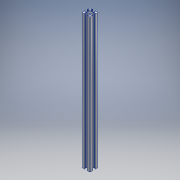
# Autodesk Inventor part: 2020 Extrusion - Double Z motor - Bed X
Saved by Autodesk Inventor 2016 (Build 200138000, 138)
## iProperties
Created: 2017-02-04
Part Number: 2020 Extrusion - Double Z motor - Bed X
Material: Aluminum 6061
Document SubType Name: Modeling
Designer: Scott
Mass: 170.679 g
Surface Area: 599.363 cm^2
Volume: 63.2146 cm^3
Density: 2.7 g/cm^3
Appearance: Aluminum - Flat
Author: Scott
Autodesk Inventor part; units mm, degrees
ref_plane "YZ Plane" through (0, 0, 0) normal (1, 0, 0) x (0, 1, 0)
ref_plane "XZ Plane" through (0, 0, 0) normal (0, 1, 0) x (-1, 0, 0)
ref_plane "XY Plane" through (0, 0, 0) normal (0, 0, 1) x (1, 0, 0)
sketch "Sketch1" plane through (0, 0, 0) normal (0, 0, 1) x (1, 0, 0)
  line L0 (-8, -10) -> (-3.2, -10)
  arc A0 (-10, -8) -> (-8, -10) centre (-8, -8) ccw
  line L1 (3.2, -10) -> (8, -10)
  line L2 (-8, 10) -> (-3.2, 10)
  line L3 (3.2, 10) -> (8, 10)
  line L4 (-10, 8) -> (-10, 3.2)
  arc A1 (-8, 10) -> (-10, 8) centre (-8, 8) ccw
  line L5 (-10, -3.2) -> (-10, -8)
  line L6 (10, 8) -> (10, 3.2)
  arc A2 (10, 8) -> (8, 10) centre (8, 8) ccw
  line L7 (10, -3.2) -> (10, -8)
  arc A3 (8, -10) -> (10, -8) centre (8, -8) ccw
  circle A4 centre (0, 0) radius 2.6
  line L8 (8.65, 4.6) -> (8.65, 3.2)
  line L9 (8.65, -3.2) -> (8.65, -4.6)
  arc A5 (8.15, -5.1) -> (8.65, -4.6) centre (8.15, -4.6) ccw
  arc A6 (8.65, 4.6) -> (8.15, 5.1) centre (8.15, 4.6) ccw
  line L10 (3.9, 2.0109) -> (3.9, -2.0109)
  arc A7 (4.4858, 3.4251) -> (3.9, 2.0109) centre (5.9, 2.0109) ccw
  line L11 (8.65, 3.2) -> (10, 3.2)
  line L12 (8.65, -3.2) -> (10, -3.2)
  line L13 (6.3678, -5.1) -> (8.15, -5.1)
  arc A8 (6.0142, -4.9536) -> (6.3678, -5.1) centre (6.3678, -4.6) ccw
  line L14 (6.3678, 5.1) -> (8.15, 5.1)
  arc A9 (6.3678, 5.1) -> (6.0142, 4.9536) centre (6.3678, 4.6) ccw
  line L15 (4.4858, 3.4251) -> (6.0142, 4.9536)
  line L16 (4.4858, -3.4251) -> (6.0142, -4.9536)
  arc A10 (3.9, -2.0109) -> (4.4858, -3.4251) centre (5.9, -2.0109) ccw
  line L17 (-4.6, 8.65) -> (-3.2, 8.65)
  line L18 (3.2, 8.65) -> (4.6, 8.65)
  arc A11 (5.1, 8.15) -> (4.6, 8.65) centre (4.6, 8.15) ccw
  arc A12 (-4.6, 8.65) -> (-5.1, 8.15) centre (-4.6, 8.15) ccw
  line L19 (-2.0109, 3.9) -> (2.0109, 3.9)
  arc A13 (-3.4251, 4.4858) -> (-2.0109, 3.9) centre (-2.0109, 5.9) ccw
  line L20 (-3.2, 8.65) -> (-3.2, 10)
  line L21 (3.2, 8.65) -> (3.2, 10)
  line L22 (5.1, 6.3678) -> (5.1, 8.15)
  arc A14 (4.9536, 6.0142) -> (5.1, 6.3678) centre (4.6, 6.3678) ccw
  line L23 (-5.1, 6.3678) -> (-5.1, 8.15)
  arc A15 (-5.1, 6.3678) -> (-4.9536, 6.0142) centre (-4.6, 6.3678) ccw
  line L24 (-3.4251, 4.4858) -> (-4.9536, 6.0142)
  line L25 (3.4251, 4.4858) -> (4.9536, 6.0142)
  arc A16 (2.0109, 3.9) -> (3.4251, 4.4858) centre (2.0109, 5.9) ccw
  line L26 (-8.65, -4.6) -> (-8.65, -3.2)
  line L27 (-8.65, 3.2) -> (-8.65, 4.6)
  arc A17 (-8.15, 5.1) -> (-8.65, 4.6) centre (-8.15, 4.6) ccw
  arc A18 (-8.65, -4.6) -> (-8.15, -5.1) centre (-8.15, -4.6) ccw
  line L28 (-3.9, -2.0109) -> (-3.9, 2.0109)
  arc A19 (-4.4858, -3.4251) -> (-3.9, -2.0109) centre (-5.9, -2.0109) ccw
  line L29 (-8.65, -3.2) -> (-10, -3.2)
  line L30 (-8.65, 3.2) -> (-10, 3.2)
  line L31 (-6.3678, 5.1) -> (-8.15, 5.1)
  arc A20 (-6.0142, 4.9536) -> (-6.3678, 5.1) centre (-6.3678, 4.6) ccw
  line L32 (-6.3678, -5.1) -> (-8.15, -5.1)
  arc A21 (-6.3678, -5.1) -> (-6.0142, -4.9536) centre (-6.3678, -4.6) ccw
  line L33 (-4.4858, -3.4251) -> (-6.0142, -4.9536)
  line L34 (-4.4858, 3.4251) -> (-6.0142, 4.9536)
  arc A22 (-3.9, 2.0109) -> (-4.4858, 3.4251) centre (-5.9, 2.0109) ccw
  line L35 (4.6, -8.65) -> (3.2, -8.65)
  line L36 (-3.2, -8.65) -> (-4.6, -8.65)
  arc A23 (-5.1, -8.15) -> (-4.6, -8.65) centre (-4.6, -8.15) ccw
  arc A24 (4.6, -8.65) -> (5.1, -8.15) centre (4.6, -8.15) ccw
  line L37 (2.0109, -3.9) -> (-2.0109, -3.9)
  arc A25 (3.4251, -4.4858) -> (2.0109, -3.9) centre (2.0109, -5.9) ccw
  line L38 (3.2, -8.65) -> (3.2, -10)
  line L39 (-3.2, -8.65) -> (-3.2, -10)
  line L40 (-5.1, -6.3678) -> (-5.1, -8.15)
  arc A26 (-4.9536, -6.0142) -> (-5.1, -6.3678) centre (-4.6, -6.3678) ccw
  line L41 (5.1, -6.3678) -> (5.1, -8.15)
  arc A27 (5.1, -6.3678) -> (4.9536, -6.0142) centre (4.6, -6.3678) ccw
  line L42 (3.4251, -4.4858) -> (4.9536, -6.0142)
  line L43 (-3.4251, -4.4858) -> (-4.9536, -6.0142)
  arc A28 (-2.0109, -3.9) -> (-3.4251, -4.4858) centre (-2.0109, -5.9) ccw
  dimension "d0" = 0.5
  dimension "d1" = 2
  dimension "d2" = 5.2
  dimension "d3" = 45
  dimension "d4" = 45
  dimension "d5" = 45
  dimension "d6" = 90
  dimension "d7" = 90
  dimension "d8" = 45
  dimension "d9" = 45
  dimension "d10" = 90
  dimension "d11" = 90
  dimension "d12" = 90
  dimension "d13" = 90
  dimension "d14" = 90
  dimension "d15" = 90
  dimension "d16" = 90
  dimension "d17" = 90
  dimension "d18" = 90
  dimension "d19" = 90
  dimension "d20" = 90
  dimension "d21" = 90
  dimension "d22" = 90
  dimension "d23" = 90
  dimension "d24" = 1.35
  dimension "d25" = 4.9
  dimension "d26" = 6.1
  dimension "d27" = 6.8
  dimension "d28" = 13.2
  dimension "d29" = 13.9
  dimension "d30" = 15.1
  dimension "d31" = 18.65
  dimension "d32" = 20
  dimension "d33" = 6.4
  dimension "d34" = 1.9
  dimension "d35" = 8.3
  dimension "d36" = 6.8
  dimension "d37" = 13.2
  dimension "d38" = 5.45
  dimension "d39" = 11.85
  dimension "d40" = 0.7
  dimension "d41" = 7.1
  dimension "d42" = 1.5
  dimension "d43" = 1.5
  dimension "d44" = 10
  dimension "d45" = 10
  dimension "d46" = 3.2
  dimension "d47" = 8.65
  dimension "d48" = 0.75
  dimension "d49" = 0.75
  dimension "d50" = 5.1
  dimension "d51" = 0.75
  dimension "d52" = 3.2
  dimension "d53" = 3.2
  dimension "d54" = 8.65
  dimension "d55" = 8.65
  dimension "d56" = 0.75
  dimension "d57" = 0.75
  dimension "d58" = 5.1
  dimension "d59" = 0.75
  dimension "d60" = 10
  dimension "d61" = 10
  dimension "d62" = 5.1
  dimension "d63" = 5.1
  constraints: 88 end point, 56 point on circle, 56 tangent, 29 centre point, 26 equal radius, 20 parallel, 1 horizontal, 1 perpendicular, 1 vertical
  measures "d0" radius of A6
  measures "d1" radius of A2
  measures "d2" diameter of A4
  measures "d3" angle of L6 L15
  measures "d4" angle of L6 L16
  measures "d5" angle of L6 L42
  measures "d6" angle of L17 L6
  measures "d7" angle of L36 L6
  measures "d8" angle of L6 L43
  measures "d9" angle of L6 L33
  measures "d10" angle of L2 L6
  measures "d11" angle of L0 L6
  measures "d12" angle of L6 L31
  measures "d13" angle of L6 L32
  measures "d14" angle of L30 L6
  measures "d15" angle of L29 L6
  measures "d16" angle of L11 L7
  measures "d17" angle of L11 L9
  measures "d18" angle of L11 L41
  measures "d19" angle of L11 L38
  measures "d20" angle of L11 L39
  measures "d21" angle of L11 L40
  measures "d22" angle of L11 L26
  measures "d23" angle of L11 L5
  measures "d24" distance between parallel lines of L8 L6
  measures "d25" distance between parallel lines of L6 L22
  measures "d26" distance between parallel lines of L6 L10
  measures "d27" distance between parallel lines of L21 L6
  measures "d28" distance between parallel lines of L20 L6
  measures "d29" distance between parallel lines of L6 L28
  measures "d30" distance between parallel lines of L6 L23
  measures "d31" distance between parallel lines of L6 L27
  measures "d32" distance between parallel lines of L6 L4
  measures "d33" distance between parallel lines of L11 L12
  measures "d34" distance between parallel lines of L11 L14
  measures "d35" distance between parallel lines of L11 L13
  measures "d36" distance between parallel lines of L11 L3
  measures "d37" distance between parallel lines of L11 L1
  measures "d38" distance between parallel lines of L11 L18
  measures "d39" distance between parallel lines of L11 L35
  measures "d40" distance between parallel lines of L11 L19
  measures "d41" distance between parallel lines of L11 L37
  measures "d42" distance between parallel lines of L25 L15
  measures "d43" distance between parallel lines of L24 L34
  measures "d44" distance from line of point (0, 0) L6
  measures "d45" distance from line of point (0, 0) L7
  measures "d46" distance from line of point (0, 0) L11
  measures "d47" distance from line of point (0, 0) L9
  measures "d48" distance from line of point (0, 0) L15
  measures "d49" distance from line of point (0, 0) L16
  measures "d50" distance from line of point (0, 0) L41
  measures "d51" distance from line of point (0, 0) L42
  measures "d52" distance from line of point (0, 0) L38
  measures "d53" distance from line of point (0, 0) L39
  measures "d54" distance from line of point (0, 0) L17
  measures "d55" distance from line of point (0, 0) L36
  measures "d56" distance from line of point (0, 0) L24
  measures "d57" distance from line of point (0, 0) L43
  measures "d58" distance from line of point (0, 0) L40
  measures "d59" distance from line of point (0, 0) L33
  measures "d60" distance from line of point (0, 0) L2
  measures "d61" distance from line of point (0, 0) L0
  measures "d62" distance from line of point (0, 0) L31
  measures "d63" distance from line of point (0, 0) L32
extrude "Extrusion1" add sketch "Sketch1" along normal mid plane 335
equation "\"platform_width\" = 214"
equation "\"platform_depth\" = 214"
equation "\"bed_cl_y_offset\" = 173.25"
body "Solid1"
